Autodesk Inventor part; units mm, degrees
(part 2 of 3)
sketch "Sketch12" plane through (0, 0, 5) normal (0, 0, 1) x (1, 0, 0)
  circle A0 centre (-43.6086, -47.5396) radius 2.1 projected
  circle A1 centre (-50.585, -18.9546) radius 2.1 projected
  circle A2 centre (-57.5615, -47.5396) radius 2.1 projected
  circle A3 centre (-85.8051, -39.2889) radius 2.1 projected
  circle A4 centre (-64.538, -59.6232) radius 2.1 projected
  circle A5 centre (-85.8051, -79.9575) radius 2.1 projected
  circle A6 centre (-57.5615, -71.7068) radius 2.1 projected
  circle A7 centre (-50.585, -100.2918) radius 2.1 projected
  circle A8 centre (-43.6086, -71.7068) radius 2.1 projected
  circle A9 centre (-15.365, -79.9575) radius 2.1 projected
  circle A10 centre (-15.365, -39.2889) radius 2.1 projected
  circle A11 centre (-36.6321, -59.6232) radius 2.1 projected
  line L0 (-44.13, -38.9303) -> (-49.053, -44.7973) projected
  arc A12 (-52.1171, -44.7973) -> (-49.053, -44.7973) centre (-50.585, -43.5117) ccw projected
  line L1 (-52.1171, -44.7973) -> (-57.0401, -38.9303) projected
  arc A13 (-55.2842, -34.0514) -> (-57.0401, -38.9303) centre (-54.742, -37.0019) ccw projected
  arc A14 (-45.8859, -34.0514) -> (-55.2842, -34.0514) centre (-50.585, -59.6232) ccw projected
  arc A15 (-44.13, -38.9303) -> (-45.8859, -34.0514) centre (-46.4281, -37.0019) ccw projected
  line L2 (-65.2781, -43.6865) -> (-62.6586, -50.8834) projected
  arc A16 (-64.1907, -53.5371) -> (-62.6586, -50.8834) centre (-64.538, -51.5674) ccw projected
  line L3 (-64.1907, -53.5371) -> (-71.7331, -54.867) projected
  arc A17 (-75.0805, -50.9068) -> (-71.7331, -54.867) centre (-72.2541, -51.9126) ccw projected
  arc A18 (-70.3813, -42.7677) -> (-75.0805, -50.9068) centre (-50.585, -59.6232) ccw projected
  arc A19 (-65.2781, -43.6865) -> (-70.3813, -42.7677) centre (-68.0971, -44.7125) ccw projected
  line L4 (-71.7331, -64.3793) -> (-64.1907, -65.7093) projected
  arc A20 (-62.6586, -68.3629) -> (-64.1907, -65.7093) centre (-64.538, -67.6789) ccw projected
  line L5 (-62.6586, -68.3629) -> (-65.2781, -75.5599) projected
  arc A21 (-70.3813, -76.4787) -> (-65.2781, -75.5599) centre (-68.0971, -74.5338) ccw projected
  arc A22 (-75.0805, -68.3395) -> (-70.3813, -76.4787) centre (-50.585, -59.6232) ccw projected
  arc A23 (-71.7331, -64.3793) -> (-75.0805, -68.3395) centre (-72.2541, -67.3338) ccw projected
  line L6 (-57.0401, -80.316) -> (-52.1171, -74.449) projected
  arc A24 (-49.053, -74.449) -> (-52.1171, -74.449) centre (-50.585, -75.7346) ccw projected
  line L7 (-49.053, -74.449) -> (-44.13, -80.316) projected
  arc A25 (-45.8859, -85.195) -> (-44.13, -80.316) centre (-46.4281, -82.2444) ccw projected
  arc A26 (-55.2842, -85.195) -> (-45.8859, -85.195) centre (-50.585, -59.6232) ccw projected
  arc A27 (-57.0401, -80.316) -> (-55.2842, -85.195) centre (-54.742, -82.2444) ccw projected
  line L8 (-35.892, -75.5599) -> (-38.5115, -68.3629) projected
  arc A28 (-36.9794, -65.7093) -> (-38.5115, -68.3629) centre (-36.6321, -67.6789) ccw projected
  line L9 (-36.9794, -65.7093) -> (-29.437, -64.3793) projected
  arc A29 (-26.0896, -68.3395) -> (-29.437, -64.3793) centre (-28.916, -67.3338) ccw projected
  arc A30 (-30.7888, -76.4787) -> (-26.0896, -68.3395) centre (-50.585, -59.6232) ccw projected
  arc A31 (-35.892, -75.5599) -> (-30.7888, -76.4787) centre (-33.073, -74.5338) ccw projected
  line L10 (-29.437, -54.867) -> (-36.9794, -53.5371) projected
  arc A32 (-38.5115, -50.8834) -> (-36.9794, -53.5371) centre (-36.6321, -51.5674) ccw projected
  line L11 (-38.5115, -50.8834) -> (-35.892, -43.6865) projected
  arc A33 (-30.7888, -42.7677) -> (-35.892, -43.6865) centre (-33.073, -44.7125) ccw projected
  arc A34 (-26.0896, -50.9068) -> (-30.7888, -42.7677) centre (-50.585, -59.6232) ccw projected
  arc A35 (-29.437, -54.867) -> (-26.0896, -50.9068) centre (-28.916, -51.9126) ccw projected
  arc A36 (-83.4142, -91.845) -> (-62.0753, -104.165) centre (-50.585, -59.6232) ccw projected
  arc A37 (-83.0768, -85.9345) -> (-83.4142, -91.845) centre (-80.5595, -89.0431) ccw projected
  line L12 (-83.0768, -85.9345) -> (-78.075, -81.8841) projected
  arc A38 (-74.0235, -82.1373) -> (-78.075, -81.8841) centre (-76.1871, -84.2156) ccw projected
  arc A39 (-74.0235, -82.1373) -> (-58.3636, -91.1786) centre (-50.585, -59.6232) ccw projected
  arc A40 (-56.1186, -94.5607) -> (-58.3636, -91.1786) centre (-59.0817, -94.0914) ccw projected
  line L13 (-56.1186, -94.5607) -> (-57.1254, -100.9175) projected
  arc A41 (-62.0753, -104.165) -> (-57.1254, -100.9175) centre (-61.0762, -100.2918) ccw projected
  arc A42 (-39.0948, -104.165) -> (-17.7559, -91.845) centre (-50.585, -59.6232) ccw projected
  arc A43 (-44.0447, -100.9175) -> (-39.0948, -104.165) centre (-40.0939, -100.2918) ccw projected
  line L14 (-44.0447, -100.9175) -> (-45.0515, -94.5607) projected
  arc A44 (-42.8065, -91.1786) -> (-45.0515, -94.5607) centre (-42.0884, -94.0914) ccw projected
  arc A45 (-42.8065, -91.1786) -> (-27.1466, -82.1373) centre (-50.585, -59.6232) ccw projected
  arc A46 (-23.0951, -81.8841) -> (-27.1466, -82.1373) centre (-24.983, -84.2156) ccw projected
  line L15 (-23.0951, -81.8841) -> (-18.0933, -85.9345) projected
  arc A47 (-17.7559, -91.845) -> (-18.0933, -85.9345) centre (-20.6106, -89.0431) ccw projected
  arc A48 (-6.2656, -71.9432) -> (-6.2656, -47.3031) centre (-50.585, -59.6232) ccw projected
  arc A49 (-11.5529, -74.6062) -> (-6.2656, -71.9432) centre (-10.1194, -70.8719) ccw projected
  line L16 (-11.5529, -74.6062) -> (-17.5615, -72.2997) projected
  arc A50 (-19.368, -68.6644) -> (-17.5615, -72.2997) centre (-16.4864, -69.499) ccw projected
  arc A51 (-19.368, -68.6644) -> (-19.368, -50.5819) centre (-50.585, -59.6232) ccw projected
  arc A52 (-17.5615, -46.9466) -> (-19.368, -50.5819) centre (-16.4864, -49.7474) ccw projected
  line L17 (-17.5615, -46.9466) -> (-11.5529, -44.6401) projected
  arc A53 (-6.2656, -47.3031) -> (-11.5529, -44.6401) centre (-10.1194, -48.3745) ccw projected
  arc A54 (-17.7559, -27.4014) -> (-39.0948, -15.0814) centre (-50.585, -59.6232) ccw projected
  arc A55 (-18.0933, -33.3119) -> (-17.7559, -27.4014) centre (-20.6106, -30.2033) ccw projected
  line L18 (-18.0933, -33.3119) -> (-23.0951, -37.3622) projected
  arc A56 (-27.1466, -37.109) -> (-23.0951, -37.3622) centre (-24.983, -35.0308) ccw projected
  arc A57 (-27.1466, -37.109) -> (-42.8065, -28.0678) centre (-50.585, -59.6232) ccw projected
  arc A58 (-45.0515, -24.6857) -> (-42.8065, -28.0678) centre (-42.0884, -25.155) ccw projected
  line L19 (-45.0515, -24.6857) -> (-44.0447, -18.3288) projected
  arc A59 (-39.0948, -15.0814) -> (-44.0447, -18.3288) centre (-40.0939, -18.9546) ccw projected
  arc A60 (-62.0753, -15.0814) -> (-83.4142, -27.4014) centre (-50.585, -59.6232) ccw projected
  arc A61 (-57.1254, -18.3288) -> (-62.0753, -15.0814) centre (-61.0762, -18.9546) ccw projected
  line L20 (-57.1254, -18.3288) -> (-56.1186, -24.6857) projected
  arc A62 (-58.3636, -28.0678) -> (-56.1186, -24.6857) centre (-59.0817, -25.155) ccw projected
  arc A63 (-58.3636, -28.0678) -> (-74.0235, -37.109) centre (-50.585, -59.6232) ccw projected
  arc A64 (-78.075, -37.3622) -> (-74.0235, -37.109) centre (-76.1871, -35.0308) ccw projected
  line L21 (-78.075, -37.3622) -> (-83.0768, -33.3119) projected
  arc A65 (-83.4142, -27.4014) -> (-83.0768, -33.3119) centre (-80.5595, -30.2033) ccw projected
  arc A66 (-94.9045, -47.3031) -> (-94.9045, -71.9432) centre (-50.585, -59.6232) ccw projected
  arc A67 (-89.6172, -44.6401) -> (-94.9045, -47.3031) centre (-91.0507, -48.3745) ccw projected
  line L22 (-89.6172, -44.6401) -> (-83.6086, -46.9466) projected
  arc A68 (-81.8021, -50.5819) -> (-83.6086, -46.9466) centre (-84.6837, -49.7474) ccw projected
  arc A69 (-81.8021, -50.5819) -> (-81.8021, -68.6644) centre (-50.585, -59.6232) ccw projected
  arc A70 (-83.6086, -72.2997) -> (-81.8021, -68.6644) centre (-84.6837, -69.499) ccw projected
  line L23 (-83.6086, -72.2997) -> (-89.6172, -74.6062) projected
  arc A71 (-94.9045, -71.9432) -> (-89.6172, -74.6062) centre (-91.0507, -70.8719) ccw projected
  circle A72 centre (-36.0848, -126.8778) radius 16 projected
  circle A73 centre (-50.585, -59.6232) radius 8 projected
  circle A74 centre (4.8498, -18.875) radius 8 projected
  circle A75 centre (-26.0687, -154.0932) radius 1.5 projected
  circle A76 centre (-104.9663, -72.7226) radius 1.5 projected
  circle A77 centre (-102.1649, -37.0532) radius 1.5 projected
  circle A78 centre (14.3857, 5.6417) radius 1.5 projected
  circle A79 centre (13.3039, -43.7854) radius 1.5 projected
  circle A80 centre (31.1494, -18.2994) radius 1.5 projected
  circle A81 centre (-15.6668, -2.4109) radius 1.5 projected
  circle A82 centre (-91.1309, -21.0881) radius 1.5 projected
  circle A83 centre (-106.5395, -53.3794) radius 1.5 projected
  circle A84 centre (-53.3702, -150.5044) radius 1.5 projected
  circle A85 centre (-7.6073, -133.6622) radius 1.5 projected
  line L24 (-9.7265, -123.6247) -> (9.9725, -47.9268) projected
  line L25 (9.9725, -47.9268) -> (17.8509, -46.5376) projected
  line L26 (17.8509, -46.5376) -> (17.2063, -42.8816) projected
  arc A86 (17.2063, -42.8816) -> (31.6348, -22.2755) centre (4.8498, -18.875) ccw projected
  line L27 (31.6348, -22.2755) -> (35.2909, -21.6308) projected
  line L28 (35.2909, -21.6308) -> (33.9017, -13.7524) projected
  line L29 (33.9017, -13.7524) -> (27.008, -14.9679) projected
  arc A87 (27.008, -14.9679) -> (16.0998, 0.6106) centre (4.8498, -18.875) ccw projected
  line L30 (16.0998, 0.6106) -> (19.5998, 6.6727) projected
  line L31 (19.5998, 6.6727) -> (12.6716, 10.6727) projected
  line L32 (12.6716, 10.6727) -> (10.8154, 7.4577) projected
  arc A88 (10.8154, 7.4577) -> (-13.4829, 0.947) centre (4.8498, -18.875) ccw projected
  line L33 (-13.4829, 0.947) -> (-16.6979, 2.8032) projected
  line L34 (-16.6979, 2.8032) -> (-20.6979, -4.125) projected
  line L35 (-20.6979, -4.125) -> (-55.4348, -7.3477) projected
  arc A89 (-55.4348, -7.3477) -> (-76.835, -14.1568) centre (-50.585, -59.6232) ccw projected
  line L36 (-76.835, -14.1568) -> (-80.3713, -8.0318) projected
  line L37 (-80.3713, -8.0318) -> (-92.9509, -17.9357) projected
  arc A90 (-92.9509, -17.9357) -> (-96.423, -21.7867) centre (-50.585, -59.6232) ccw projected
  line L38 (-96.423, -21.7867) -> (-95.6743, -22.4047) projected
  arc A91 (-95.3624, -25.1669) -> (-95.6743, -22.4047) centre (-96.9475, -23.9472) ccw projected
  arc A92 (-95.3624, -25.1669) -> (-100.1355, -32.4754) centre (-50.585, -59.6232) ccw projected
  arc A93 (-102.79, -33.3003) -> (-100.1355, -32.4754) centre (-101.8895, -31.5145) ccw projected
  line L39 (-102.79, -33.3003) -> (-103.9829, -32.6988) projected
  arc A94 (-103.9829, -32.6988) -> (-106.5047, -38.4279) centre (-50.585, -59.6232) ccw projected
  line L40 (-106.5047, -38.4279) -> (-109.6106, -50.019) projected
  arc A95 (-109.6106, -50.019) -> (-110.2911, -56.2415) centre (-50.585, -59.6232) ccw projected
  line L41 (-110.2911, -56.2415) -> (-108.9573, -56.317) projected
  arc A96 (-107.0709, -58.3586) -> (-108.9573, -56.317) centre (-109.0704, -58.3138) ccw projected
  arc A97 (-107.0709, -58.3586) -> (-106.5915, -67.0745) centre (-50.585, -59.6232) ccw projected
  arc A98 (-108.2427, -69.3107) -> (-106.5915, -67.0745) centre (-108.5741, -67.3383) ccw projected
  line L42 (-108.2427, -69.3107) -> (-109.2001, -69.4715) projected
  arc A99 (-109.2001, -69.4715) -> (-108.1187, -74.5427) centre (-50.585, -59.6232) ccw projected
  line L43 (-108.1187, -74.5427) -> (-102.1764, -89.4094) projected
  line L44 (-102.1764, -89.4094) -> (-96.0514, -85.8732) projected
  arc A100 (-96.0514, -85.8732) -> (-93.2051, -90.2791) centre (-50.585, -59.6232) ccw projected
  line L45 (-93.2051, -90.2791) -> (-56.6733, -141.0681) projected
  arc A101 (-57.2313, -148.7428) -> (-56.6733, -141.0681) centre (-61.5442, -144.5716) ccw projected
  line L46 (-57.2313, -148.7428) -> (-59.0263, -150.5988) projected
  line L47 (-59.0263, -150.5988) -> (-54.7134, -154.77) projected
  line L48 (-54.7134, -154.77) -> (-51.8854, -154.7228) projected
  line L49 (-51.8854, -154.7228) -> (-50.3657, -153.1515) projected
  arc A102 (-48.0859, -152.7278) -> (-50.3657, -153.1515) centre (-48.9281, -154.5419) ccw projected
  arc A103 (-48.0859, -152.7278) -> (-31.6953, -155.0377) centre (-36.0848, -126.8778) ccw projected
  arc A104 (-29.5104, -156.3231) -> (-31.6953, -155.0377) centre (-31.3873, -157.0139) ccw projected
  line L50 (-29.5104, -156.3231) -> (-29.1318, -157.3516) projected
  line L51 (-29.1318, -157.3516) -> (-26.5641, -158.5378) projected
  line L52 (-26.5641, -158.5378) -> (-22.8103, -157.1563) projected
  line L53 (-22.8103, -157.1563) -> (-21.6241, -154.5886) projected
  line L54 (-21.6241, -154.5886) -> (-22.0027, -153.56) projected
  arc A105 (-21.1722, -151.1649) -> (-22.0027, -153.56) centre (-20.1257, -152.8693) ccw projected
  arc A106 (-21.1722, -151.1649) -> (-10.1895, -138.7808) centre (-36.0848, -126.8778) ccw projected
  arc A107 (-8.179, -137.6255) -> (-10.1895, -138.7808) centre (-8.3723, -139.6161) ccw projected
  line L55 (-8.179, -137.6255) -> (-6.0033, -137.8368) projected
  line L56 (-6.0033, -137.8368) -> (-3.8193, -136.0394) projected
  line L57 (-3.8193, -136.0394) -> (-3.2394, -130.0675) projected
  line L58 (-3.2394, -130.0675) -> (-5.371, -129.8605) projected
  arc A108 (-9.7265, -123.6247) -> (-5.371, -129.8605) centre (-4.8877, -124.8839) ccw projected
  circle A109 centre (-26.0687, -154.0932) radius 1.5 projected
  line L59 (-36.0848, -126.8778) -> (-26.0687, -154.0932)
  line L60 (-36.0848, -126.8778) -> (-45.311, -146.8497)
  circle A110 centre (-45.311, -146.8497) radius 2.05
  point P0 (0, 0)
  dimension "d80" = 22
  dimension "d81" = 45
  dimension "d82" = 4.1
  constraints: 4 end point, 1 centre point, 1 coincident
  measures "d80" distance of L59.start L60.end
  measures "d81" angle of L59 L60
  measures "d82" diameter of A110
extrude "Extrusion11" cut sketch "Sketch12" against normal blind 10 contours A110
pattern_circular "Circular Pattern6" count 4 over 360 about axis through (-36.0848, -126.8778, 5) along (0, 0, -1) of "Extrusion11"
sketch "Sketch13" plane through (0, 0, 5) normal (0, 0, 1) x (1, 0, 0)
  circle A0 centre (-16.1129, -136.1039) radius 2.05 projected
  circle A1 centre (-26.8587, -106.9059) radius 2.05 projected
  circle A2 centre (-56.0568, -117.6516) radius 2.05 projected
  circle A3 centre (-45.311, -146.8497) radius 2.05 projected
  circle A4 centre (-43.6086, -47.5396) radius 2.1 projected
  circle A5 centre (-50.585, -18.9546) radius 2.1 projected
  circle A6 centre (-57.5615, -47.5396) radius 2.1 projected
  circle A7 centre (-85.8051, -39.2889) radius 2.1 projected
  circle A8 centre (-64.538, -59.6232) radius 2.1 projected
  circle A9 centre (-85.8051, -79.9575) radius 2.1 projected
  circle A10 centre (-57.5615, -71.7068) radius 2.1 projected
  circle A11 centre (-50.585, -100.2918) radius 2.1 projected
  circle A12 centre (-43.6086, -71.7068) radius 2.1 projected
  circle A13 centre (-15.365, -79.9575) radius 2.1 projected
  circle A14 centre (-15.365, -39.2889) radius 2.1 projected
  circle A15 centre (-36.6321, -59.6232) radius 2.1 projected
  line L0 (-44.13, -38.9303) -> (-49.053, -44.7973) projected
  arc A16 (-52.1171, -44.7973) -> (-49.053, -44.7973) centre (-50.585, -43.5117) ccw projected
  line L1 (-52.1171, -44.7973) -> (-57.0401, -38.9303) projected
  arc A17 (-55.2842, -34.0514) -> (-57.0401, -38.9303) centre (-54.742, -37.0019) ccw projected
  arc A18 (-45.8859, -34.0514) -> (-55.2842, -34.0514) centre (-50.585, -59.6232) ccw projected
  arc A19 (-44.13, -38.9303) -> (-45.8859, -34.0514) centre (-46.4281, -37.0019) ccw projected
  line L2 (-65.2781, -43.6865) -> (-62.6586, -50.8834) projected
  arc A20 (-64.1907, -53.5371) -> (-62.6586, -50.8834) centre (-64.538, -51.5674) ccw projected
  line L3 (-64.1907, -53.5371) -> (-71.7331, -54.867) projected
  arc A21 (-75.0805, -50.9068) -> (-71.7331, -54.867) centre (-72.2541, -51.9126) ccw projected
  arc A22 (-70.3813, -42.7677) -> (-75.0805, -50.9068) centre (-50.585, -59.6232) ccw projected
  arc A23 (-65.2781, -43.6865) -> (-70.3813, -42.7677) centre (-68.0971, -44.7125) ccw projected
  line L4 (-71.7331, -64.3793) -> (-64.1907, -65.7093) projected
  arc A24 (-62.6586, -68.3629) -> (-64.1907, -65.7093) centre (-64.538, -67.6789) ccw projected
  line L5 (-62.6586, -68.3629) -> (-65.2781, -75.5599) projected
  arc A25 (-70.3813, -76.4787) -> (-65.2781, -75.5599) centre (-68.0971, -74.5338) ccw projected
  arc A26 (-75.0805, -68.3395) -> (-70.3813, -76.4787) centre (-50.585, -59.6232) ccw projected
  arc A27 (-71.7331, -64.3793) -> (-75.0805, -68.3395) centre (-72.2541, -67.3338) ccw projected
  line L6 (-57.0401, -80.316) -> (-52.1171, -74.449) projected
  arc A28 (-49.053, -74.449) -> (-52.1171, -74.449) centre (-50.585, -75.7346) ccw projected
  line L7 (-49.053, -74.449) -> (-44.13, -80.316) projected
  arc A29 (-45.8859, -85.195) -> (-44.13, -80.316) centre (-46.4281, -82.2444) ccw projected
  arc A30 (-55.2842, -85.195) -> (-45.8859, -85.195) centre (-50.585, -59.6232) ccw projected
  arc A31 (-57.0401, -80.316) -> (-55.2842, -85.195) centre (-54.742, -82.2444) ccw projected
  line L8 (-35.892, -75.5599) -> (-38.5115, -68.3629) projected
  arc A32 (-36.9794, -65.7093) -> (-38.5115, -68.3629) centre (-36.6321, -67.6789) ccw projected
  line L9 (-36.9794, -65.7093) -> (-29.437, -64.3793) projected
  arc A33 (-26.0896, -68.3395) -> (-29.437, -64.3793) centre (-28.916, -67.3338) ccw projected
  arc A34 (-30.7888, -76.4787) -> (-26.0896, -68.3395) centre (-50.585, -59.6232) ccw projected
  arc A35 (-35.892, -75.5599) -> (-30.7888, -76.4787) centre (-33.073, -74.5338) ccw projected
  line L10 (-29.437, -54.867) -> (-36.9794, -53.5371) projected
  arc A36 (-38.5115, -50.8834) -> (-36.9794, -53.5371) centre (-36.6321, -51.5674) ccw projected
  line L11 (-38.5115, -50.8834) -> (-35.892, -43.6865) projected
  arc A37 (-30.7888, -42.7677) -> (-35.892, -43.6865) centre (-33.073, -44.7125) ccw projected
  arc A38 (-26.0896, -50.9068) -> (-30.7888, -42.7677) centre (-50.585, -59.6232) ccw projected
  arc A39 (-29.437, -54.867) -> (-26.0896, -50.9068) centre (-28.916, -51.9126) ccw projected
  arc A40 (-83.4142, -91.845) -> (-62.0753, -104.165) centre (-50.585, -59.6232) ccw projected
  arc A41 (-83.0768, -85.9345) -> (-83.4142, -91.845) centre (-80.5595, -89.0431) ccw projected
  line L12 (-83.0768, -85.9345) -> (-78.075, -81.8841) projected
  arc A42 (-74.0235, -82.1373) -> (-78.075, -81.8841) centre (-76.1871, -84.2156) ccw projected
  arc A43 (-74.0235, -82.1373) -> (-58.3636, -91.1786) centre (-50.585, -59.6232) ccw projected
  arc A44 (-56.1186, -94.5607) -> (-58.3636, -91.1786) centre (-59.0817, -94.0914) ccw projected
  line L13 (-56.1186, -94.5607) -> (-57.1254, -100.9175) projected
  arc A45 (-62.0753, -104.165) -> (-57.1254, -100.9175) centre (-61.0762, -100.2918) ccw projected
  arc A46 (-39.0948, -104.165) -> (-17.7559, -91.845) centre (-50.585, -59.6232) ccw projected
  arc A47 (-44.0447, -100.9175) -> (-39.0948, -104.165) centre (-40.0939, -100.2918) ccw projected
  line L14 (-44.0447, -100.9175) -> (-45.0515, -94.5607) projected
  arc A48 (-42.8065, -91.1786) -> (-45.0515, -94.5607) centre (-42.0884, -94.0914) ccw projected
  arc A49 (-42.8065, -91.1786) -> (-27.1466, -82.1373) centre (-50.585, -59.6232) ccw projected
  arc A50 (-23.0951, -81.8841) -> (-27.1466, -82.1373) centre (-24.983, -84.2156) ccw projected
  line L15 (-23.0951, -81.8841) -> (-18.0933, -85.9345) projected
  arc A51 (-17.7559, -91.845) -> (-18.0933, -85.9345) centre (-20.6106, -89.0431) ccw projected
  arc A52 (-6.2656, -71.9432) -> (-6.2656, -47.3031) centre (-50.585, -59.6232) ccw projected
  arc A53 (-11.5529, -74.6062) -> (-6.2656, -71.9432) centre (-10.1194, -70.8719) ccw projected
  line L16 (-11.5529, -74.6062) -> (-17.5615, -72.2997) projected
  arc A54 (-19.368, -68.6644) -> (-17.5615, -72.2997) centre (-16.4864, -69.499) ccw projected
  arc A55 (-19.368, -68.6644) -> (-19.368, -50.5819) centre (-50.585, -59.6232) ccw projected
  arc A56 (-17.5615, -46.9466) -> (-19.368, -50.5819) centre (-16.4864, -49.7474) ccw projected
  line L17 (-17.5615, -46.9466) -> (-11.5529, -44.6401) projected
  arc A57 (-6.2656, -47.3031) -> (-11.5529, -44.6401) centre (-10.1194, -48.3745) ccw projected
  arc A58 (-17.7559, -27.4014) -> (-39.0948, -15.0814) centre (-50.585, -59.6232) ccw projected
  arc A59 (-18.0933, -33.3119) -> (-17.7559, -27.4014) centre (-20.6106, -30.2033) ccw projected
  line L18 (-18.0933, -33.3119) -> (-23.0951, -37.3622) projected
  arc A60 (-27.1466, -37.109) -> (-23.0951, -37.3622) centre (-24.983, -35.0308) ccw projected
  arc A61 (-27.1466, -37.109) -> (-42.8065, -28.0678) centre (-50.585, -59.6232) ccw projected
  arc A62 (-45.0515, -24.6857) -> (-42.8065, -28.0678) centre (-42.0884, -25.155) ccw projected
  line L19 (-45.0515, -24.6857) -> (-44.0447, -18.3288) projected
  arc A63 (-39.0948, -15.0814) -> (-44.0447, -18.3288) centre (-40.0939, -18.9546) ccw projected
  arc A64 (-62.0753, -15.0814) -> (-83.4142, -27.4014) centre (-50.585, -59.6232) ccw projected
  arc A65 (-57.1254, -18.3288) -> (-62.0753, -15.0814) centre (-61.0762, -18.9546) ccw projected
  line L20 (-57.1254, -18.3288) -> (-56.1186, -24.6857) projected
  arc A66 (-58.3636, -28.0678) -> (-56.1186, -24.6857) centre (-59.0817, -25.155) ccw projected
  arc A67 (-58.3636, -28.0678) -> (-74.0235, -37.109) centre (-50.585, -59.6232) ccw projected
  arc A68 (-78.075, -37.3622) -> (-74.0235, -37.109) centre (-76.1871, -35.0308) ccw projected
  line L21 (-78.075, -37.3622) -> (-83.0768, -33.3119) projected
  arc A69 (-83.4142, -27.4014) -> (-83.0768, -33.3119) centre (-80.5595, -30.2033) ccw projected
  arc A70 (-94.9045, -47.3031) -> (-94.9045, -71.9432) centre (-50.585, -59.6232) ccw projected
  arc A71 (-89.6172, -44.6401) -> (-94.9045, -47.3031) centre (-91.0507, -48.3745) ccw projected
  line L22 (-89.6172, -44.6401) -> (-83.6086, -46.9466) projected
  arc A72 (-81.8021, -50.5819) -> (-83.6086, -46.9466) centre (-84.6837, -49.7474) ccw projected
  arc A73 (-81.8021, -50.5819) -> (-81.8021, -68.6644) centre (-50.585, -59.6232) ccw projected
  arc A74 (-83.6086, -72.2997) -> (-81.8021, -68.6644) centre (-84.6837, -69.499) ccw projected
  line L23 (-83.6086, -72.2997) -> (-89.6172, -74.6062) projected
  arc A75 (-94.9045, -71.9432) -> (-89.6172, -74.6062) centre (-91.0507, -70.8719) ccw projected
  circle A76 centre (-36.0848, -126.8778) radius 16 projected
  circle A77 centre (-50.585, -59.6232) radius 8 projected
  circle A78 centre (4.8498, -18.875) radius 8 projected
  circle A79 centre (-26.0687, -154.0932) radius 1.5 projected
  circle A80 centre (-104.9663, -72.7226) radius 1.5 projected
  circle A81 centre (-102.1649, -37.0532) radius 1.5 projected
  circle A82 centre (14.3857, 5.6417) radius 1.5 projected
  circle A83 centre (13.3039, -43.7854) radius 1.5 projected
  circle A84 centre (31.1494, -18.2994) radius 1.5 projected
  circle A85 centre (-15.6668, -2.4109) radius 1.5 projected
  circle A86 centre (-91.1309, -21.0881) radius 1.5 projected
  circle A87 centre (-106.5395, -53.3794) radius 1.5 projected
  circle A88 centre (-53.3702, -150.5044) radius 1.5 projected
  circle A89 centre (-7.6073, -133.6622) radius 1.5 projected
  line L24 (-9.7265, -123.6247) -> (9.9725, -47.9268) projected
  line L25 (9.9725, -47.9268) -> (17.8509, -46.5376) projected
  line L26 (17.8509, -46.5376) -> (17.2063, -42.8816) projected
  arc A90 (17.2063, -42.8816) -> (31.6348, -22.2755) centre (4.8498, -18.875) ccw projected
  line L27 (31.6348, -22.2755) -> (35.2909, -21.6308) projected
  line L28 (35.2909, -21.6308) -> (33.9017, -13.7524) projected
  line L29 (33.9017, -13.7524) -> (27.008, -14.9679) projected
  arc A91 (27.008, -14.9679) -> (16.0998, 0.6106) centre (4.8498, -18.875) ccw projected
  line L30 (16.0998, 0.6106) -> (19.5998, 6.6727) projected
  line L31 (19.5998, 6.6727) -> (12.6716, 10.6727) projected
  line L32 (12.6716, 10.6727) -> (10.8154, 7.4577) projected
  arc A92 (10.8154, 7.4577) -> (-13.4829, 0.947) centre (4.8498, -18.875) ccw projected
  line L33 (-13.4829, 0.947) -> (-16.6979, 2.8032) projected
  line L34 (-16.6979, 2.8032) -> (-20.6979, -4.125) projected
  line L35 (-20.6979, -4.125) -> (-55.4348, -7.3477) projected
  arc A93 (-55.4348, -7.3477) -> (-76.835, -14.1568) centre (-50.585, -59.6232) ccw projected
  line L36 (-76.835, -14.1568) -> (-80.3713, -8.0318) projected
  line L37 (-80.3713, -8.0318) -> (-92.9509, -17.9357) projected
  arc A94 (-92.9509, -17.9357) -> (-96.423, -21.7867) centre (-50.585, -59.6232) ccw projected
  line L38 (-96.423, -21.7867) -> (-95.6743, -22.4047) projected
  arc A95 (-95.3624, -25.1669) -> (-95.6743, -22.4047) centre (-96.9475, -23.9472) ccw projected
  arc A96 (-95.3624, -25.1669) -> (-100.1355, -32.4754) centre (-50.585, -59.6232) ccw projected
  arc A97 (-102.79, -33.3003) -> (-100.1355, -32.4754) centre (-101.8895, -31.5145) ccw projected
  line L39 (-102.79, -33.3003) -> (-103.9829, -32.6988) projected
  arc A98 (-103.9829, -32.6988) -> (-106.5047, -38.4279) centre (-50.585, -59.6232) ccw projected
  line L40 (-106.5047, -38.4279) -> (-109.6106, -50.019) projected
  arc A99 (-109.6106, -50.019) -> (-110.2911, -56.2415) centre (-50.585, -59.6232) ccw projected
  line L41 (-110.2911, -56.2415) -> (-108.9573, -56.317) projected
  arc A100 (-107.0709, -58.3586) -> (-108.9573, -56.317) centre (-109.0704, -58.3138) ccw projected
  arc A101 (-107.0709, -58.3586) -> (-106.5915, -67.0745) centre (-50.585, -59.6232) ccw projected
  arc A102 (-108.2427, -69.3107) -> (-106.5915, -67.0745) centre (-108.5741, -67.3383) ccw projected
  line L42 (-108.2427, -69.3107) -> (-109.2001, -69.4715) projected
  arc A103 (-109.2001, -69.4715) -> (-108.1187, -74.5427) centre (-50.585, -59.6232) ccw projected
  line L43 (-108.1187, -74.5427) -> (-102.1764, -89.4094) projected
  line L44 (-102.1764, -89.4094) -> (-96.0514, -85.8732) projected
  arc A104 (-96.0514, -85.8732) -> (-93.2051, -90.2791) centre (-50.585, -59.6232) ccw projected
  line L45 (-93.2051, -90.2791) -> (-56.6733, -141.0681) projected
  arc A105 (-57.2313, -148.7428) -> (-56.6733, -141.0681) centre (-61.5442, -144.5716) ccw projected
  line L46 (-57.2313, -148.7428) -> (-59.0263, -150.5988) projected
  line L47 (-59.0263, -150.5988) -> (-54.7134, -154.77) projected
  line L48 (-54.7134, -154.77) -> (-51.8854, -154.7228) projected
  line L49 (-51.8854, -154.7228) -> (-50.3657, -153.1515) projected
  arc A106 (-48.0859, -152.7278) -> (-50.3657, -153.1515) centre (-48.9281, -154.5419) ccw projected
  arc A107 (-48.0859, -152.7278) -> (-31.6953, -155.0377) centre (-36.0848, -126.8778) ccw projected
  arc A108 (-29.5104, -156.3231) -> (-31.6953, -155.0377) centre (-31.3873, -157.0139) ccw projected
  line L50 (-29.5104, -156.3231) -> (-29.1318, -157.3516) projected
  line L51 (-29.1318, -157.3516) -> (-26.5641, -158.5378) projected
  line L52 (-26.5641, -158.5378) -> (-22.8103, -157.1563) projected
  line L53 (-22.8103, -157.1563) -> (-21.6241, -154.5886) projected
  line L54 (-21.6241, -154.5886) -> (-22.0027, -153.56) projected
  arc A109 (-21.1722, -151.1649) -> (-22.0027, -153.56) centre (-20.1257, -152.8693) ccw projected
  arc A110 (-21.1722, -151.1649) -> (-10.1895, -138.7808) centre (-36.0848, -126.8778) ccw projected
  arc A111 (-8.179, -137.6255) -> (-10.1895, -138.7808) centre (-8.3723, -139.6161) ccw projected
  line L55 (-8.179, -137.6255) -> (-6.0033, -137.8368) projected
  line L56 (-6.0033, -137.8368) -> (-3.8193, -136.0394) projected
  line L57 (-3.8193, -136.0394) -> (-3.2394, -130.0675) projected
  line L58 (-3.2394, -130.0675) -> (-5.371, -129.8605) projected
  arc A112 (-9.7265, -123.6247) -> (-5.371, -129.8605) centre (-4.8877, -124.8839) ccw projected
  line L59 (-14.8426, -119.4603) -> (-6.4101, -87.0562)
  circle A113 centre (-36.0848, -126.8778) radius 22.5
  circle A114 centre (-50.585, -59.6232) radius 52
  line L60 (-20.7537, -110.4094) -> (-18.1052, -100.2318)
  line L61 (-58.5466, -128.1884) -> (-74.7431, -105.6708)
  circle A115 centre (-36.0848, -126.8778) radius 27.5
  point P0 (0, 0)
  point P1 (-63.1181, -121.8328)
  point P2 (-58.5453, -111.0103)
  point P3 (-19.3588, -105.0491)
  point P4 (-12.9173, -112.0618)
  dimension "d88" = 45
  dimension "d89" = 6
  dimension "d90" = 104
  dimension "d91" = 8
  dimension "d92" = 6
  dimension "d93" = 55
  constraints: 6 end point, 6 point on circle, 3 centre point, 3 coincident, 3 parallel
  measures "d88" diameter of A113
  measures "d89" distance between parallel lines of L24 L59
  measures "d90" diameter of A114
  measures "d91" distance between parallel lines of L59 L60
  measures "d92" distance between parallel lines of L45 L61
  measures "d93" diameter of A115
extrude "Extrusion12" cut sketch "Sketch13" against normal blind 10 contours A115 L60 A114 L59 | L61 A114 A115
fillet "Fillet12" radius 2 5 edges at (-6.4101, -87.0562, 2.5) (-12.9173, -112.0618, 2.5) (-74.7431, -105.6708, 2.5) (-63.1181, -121.8328, 2.5) (-58.5453, -111.0103, 2.5)
fillet "Fillet13" radius 3 1 edges at (-19.3588, -105.0491, 2.5)
fillet "Fillet14" radius 5 1 edges at (-18.1052, -100.2318, 2.5)
thicken "Thicken1" operation add thickness 3 both sides no extend neighbours yes toward (-0.745193, -0.6668488, 0) faces at (-15.592, -108.5394, 1.6667)
sketch "Sketch14" plane through (0, 0, 5) normal (0, 0, 1) x (1, 0, 0)
  circle A0 centre (2.1523, -31.0805) radius 2.1 projected
  circle A1 centre (17.0553, -21.5725) radius 2.1 projected
  circle A2 centre (7.5473, -6.6695) radius 2.1 projected
  circle A3 centre (-7.3556, -16.1775) radius 2.1 projected
  point P0 (0, 0)
hole "Hole3" at (17.0553, -21.5725, 5) at (2.1523, -31.0805, 5) at (-7.3556, -16.1775, 5) at (7.5473, -6.6695, 5) direction (0, 0, -1) diameter 3.1 depth 17
sketch "Sketch15" plane through (0, 0, 5) normal (0, 0, 1) x (1, 0, 0)
  circle A0 centre (-7.3556, -16.1775) radius 1.55 projected
  circle A1 centre (17.0553, -21.5725) radius 1.55 projected
  circle A2 centre (2.1523, -31.0805) radius 1.55 projected
  circle A3 centre (7.5473, -6.6695) radius 1.55 projected
  line L0 (-8.9194, -96.699) -> (-12.8137, -111.6638) projected
  arc A4 (-16.3595, -112.3464) -> (-12.8137, -111.6638) centre (-14.7493, -111.1602) ccw projected
  arc A5 (-16.3595, -112.3464) -> (-18.9305, -109.3855) centre (-36.0848, -126.8778) ccw projected
  arc A6 (-19.7333, -106.4881) -> (-18.9305, -109.3855) centre (-16.83, -107.2436) ccw projected
  line L1 (-19.7333, -106.4881) -> (-18.513, -101.7988) projected
  arc A7 (-16.9119, -99.2479) -> (-18.513, -101.7988) centre (-13.6742, -103.058) ccw projected
  arc A8 (-16.9119, -99.2479) -> (-12.3264, -94.8408) centre (-50.585, -59.6232) ccw projected
  arc A9 (-8.9194, -96.699) -> (-12.3264, -94.8408) centre (-10.8549, -96.1953) ccw projected
  arc A10 (-68.172, -108.5588) -> (-61.3963, -110.4869) centre (-50.585, -59.6232) ccw projected
  arc A11 (-60.0679, -113.4218) -> (-61.3963, -110.4869) centre (-61.8121, -112.4432) ccw projected
  arc A12 (-60.0679, -113.4218) -> (-62.0734, -117.8863) centre (-36.0848, -126.8778) ccw projected
  arc A13 (-65.5871, -118.4003) -> (-62.0734, -117.8863) centre (-63.9634, -117.2324) ccw projected
  line L2 (-65.5871, -118.4003) -> (-70.472, -111.6088) projected
  arc A14 (-68.172, -108.5588) -> (-70.472, -111.6088) centre (-68.8484, -110.441) ccw projected
  circle A15 centre (-16.1129, -136.1039) radius 2.05 projected
  circle A16 centre (-26.8587, -106.9059) radius 2.05 projected
  circle A17 centre (-56.0568, -117.6516) radius 2.05 projected
  circle A18 centre (-45.311, -146.8497) radius 2.05 projected
  circle A19 centre (-43.6086, -47.5396) radius 2.1 projected
  circle A20 centre (-50.585, -18.9546) radius 2.1 projected
  circle A21 centre (-57.5615, -47.5396) radius 2.1 projected
  circle A22 centre (-85.8051, -39.2889) radius 2.1 projected
  circle A23 centre (-64.538, -59.6232) radius 2.1 projected
  circle A24 centre (-85.8051, -79.9575) radius 2.1 projected
  circle A25 centre (-57.5615, -71.7068) radius 2.1 projected
  circle A26 centre (-50.585, -100.2918) radius 2.1 projected
  circle A27 centre (-43.6086, -71.7068) radius 2.1 projected
  circle A28 centre (-15.365, -79.9575) radius 2.1 projected
  circle A29 centre (-15.365, -39.2889) radius 2.1 projected
  circle A30 centre (-36.6321, -59.6232) radius 2.1 projected
  line L3 (-44.13, -38.9303) -> (-49.053, -44.7973) projected
  arc A31 (-52.1171, -44.7973) -> (-49.053, -44.7973) centre (-50.585, -43.5117) ccw projected
  line L4 (-52.1171, -44.7973) -> (-57.0401, -38.9303) projected
  arc A32 (-55.2842, -34.0514) -> (-57.0401, -38.9303) centre (-54.742, -37.0019) ccw projected
  arc A33 (-45.8859, -34.0514) -> (-55.2842, -34.0514) centre (-50.585, -59.6232) ccw projected
  arc A34 (-44.13, -38.9303) -> (-45.8859, -34.0514) centre (-46.4281, -37.0019) ccw projected
  line L5 (-65.2781, -43.6865) -> (-62.6586, -50.8834) projected
  arc A35 (-64.1907, -53.5371) -> (-62.6586, -50.8834) centre (-64.538, -51.5674) ccw projected
  line L6 (-64.1907, -53.5371) -> (-71.7331, -54.867) projected
  arc A36 (-75.0805, -50.9068) -> (-71.7331, -54.867) centre (-72.2541, -51.9126) ccw projected
  arc A37 (-70.3813, -42.7677) -> (-75.0805, -50.9068) centre (-50.585, -59.6232) ccw projected
  arc A38 (-65.2781, -43.6865) -> (-70.3813, -42.7677) centre (-68.0971, -44.7125) ccw projected
  line L7 (-71.7331, -64.3793) -> (-64.1907, -65.7093) projected
  arc A39 (-62.6586, -68.3629) -> (-64.1907, -65.7093) centre (-64.538, -67.6789) ccw projected
  line L8 (-62.6586, -68.3629) -> (-65.2781, -75.5599) projected
  arc A40 (-70.3813, -76.4787) -> (-65.2781, -75.5599) centre (-68.0971, -74.5338) ccw projected
  arc A41 (-75.0805, -68.3395) -> (-70.3813, -76.4787) centre (-50.585, -59.6232) ccw projected
  arc A42 (-71.7331, -64.3793) -> (-75.0805, -68.3395) centre (-72.2541, -67.3338) ccw projected
  line L9 (-57.0401, -80.316) -> (-52.1171, -74.449) projected
  arc A43 (-49.053, -74.449) -> (-52.1171, -74.449) centre (-50.585, -75.7346) ccw projected
  line L10 (-49.053, -74.449) -> (-44.13, -80.316) projected
  arc A44 (-45.8859, -85.195) -> (-44.13, -80.316) centre (-46.4281, -82.2444) ccw projected
  arc A45 (-55.2842, -85.195) -> (-45.8859, -85.195) centre (-50.585, -59.6232) ccw projected
  arc A46 (-57.0401, -80.316) -> (-55.2842, -85.195) centre (-54.742, -82.2444) ccw projected
  line L11 (-35.892, -75.5599) -> (-38.5115, -68.3629) projected
  arc A47 (-36.9794, -65.7093) -> (-38.5115, -68.3629) centre (-36.6321, -67.6789) ccw projected
  line L12 (-36.9794, -65.7093) -> (-29.437, -64.3793) projected
  arc A48 (-26.0896, -68.3395) -> (-29.437, -64.3793) centre (-28.916, -67.3338) ccw projected
  arc A49 (-30.7888, -76.4787) -> (-26.0896, -68.3395) centre (-50.585, -59.6232) ccw projected
  arc A50 (-35.892, -75.5599) -> (-30.7888, -76.4787) centre (-33.073, -74.5338) ccw projected
  line L13 (-29.437, -54.867) -> (-36.9794, -53.5371) projected
  arc A51 (-38.5115, -50.8834) -> (-36.9794, -53.5371) centre (-36.6321, -51.5674) ccw projected
  line L14 (-38.5115, -50.8834) -> (-35.892, -43.6865) projected
  arc A52 (-30.7888, -42.7677) -> (-35.892, -43.6865) centre (-33.073, -44.7125) ccw projected
  arc A53 (-26.0896, -50.9068) -> (-30.7888, -42.7677) centre (-50.585, -59.6232) ccw projected
  arc A54 (-29.437, -54.867) -> (-26.0896, -50.9068) centre (-28.916, -51.9126) ccw projected
  arc A55 (-83.4142, -91.845) -> (-62.0753, -104.165) centre (-50.585, -59.6232) ccw projected
  arc A56 (-83.0768, -85.9345) -> (-83.4142, -91.845) centre (-80.5595, -89.0431) ccw projected
  line L15 (-83.0768, -85.9345) -> (-78.075, -81.8841) projected
  arc A57 (-74.0235, -82.1373) -> (-78.075, -81.8841) centre (-76.1871, -84.2156) ccw projected
  arc A58 (-74.0235, -82.1373) -> (-58.3636, -91.1786) centre (-50.585, -59.6232) ccw projected
  arc A59 (-56.1186, -94.5607) -> (-58.3636, -91.1786) centre (-59.0817, -94.0914) ccw projected
  line L16 (-56.1186, -94.5607) -> (-57.1254, -100.9175) projected
  arc A60 (-62.0753, -104.165) -> (-57.1254, -100.9175) centre (-61.0762, -100.2918) ccw projected
  arc A61 (-39.0948, -104.165) -> (-17.7559, -91.845) centre (-50.585, -59.6232) ccw projected
  arc A62 (-44.0447, -100.9175) -> (-39.0948, -104.165) centre (-40.0939, -100.2918) ccw projected
  line L17 (-44.0447, -100.9175) -> (-45.0515, -94.5607) projected
  arc A63 (-42.8065, -91.1786) -> (-45.0515, -94.5607) centre (-42.0884, -94.0914) ccw projected
  arc A64 (-42.8065, -91.1786) -> (-27.1466, -82.1373) centre (-50.585, -59.6232) ccw projected
  arc A65 (-23.0951, -81.8841) -> (-27.1466, -82.1373) centre (-24.983, -84.2156) ccw projected
  line L18 (-23.0951, -81.8841) -> (-18.0933, -85.9345) projected
  arc A66 (-17.7559, -91.845) -> (-18.0933, -85.9345) centre (-20.6106, -89.0431) ccw projected
  arc A67 (-6.2656, -71.9432) -> (-6.2656, -47.3031) centre (-50.585, -59.6232) ccw projected
  arc A68 (-11.5529, -74.6062) -> (-6.2656, -71.9432) centre (-10.1194, -70.8719) ccw projected
  line L19 (-11.5529, -74.6062) -> (-17.5615, -72.2997) projected
  arc A69 (-19.368, -68.6644) -> (-17.5615, -72.2997) centre (-16.4864, -69.499) ccw projected
  arc A70 (-19.368, -68.6644) -> (-19.368, -50.5819) centre (-50.585, -59.6232) ccw projected
  arc A71 (-17.5615, -46.9466) -> (-19.368, -50.5819) centre (-16.4864, -49.7474) ccw projected
  line L20 (-17.5615, -46.9466) -> (-11.5529, -44.6401) projected
  arc A72 (-6.2656, -47.3031) -> (-11.5529, -44.6401) centre (-10.1194, -48.3745) ccw projected
  arc A73 (-17.7559, -27.4014) -> (-39.0948, -15.0814) centre (-50.585, -59.6232) ccw projected
  arc A74 (-18.0933, -33.3119) -> (-17.7559, -27.4014) centre (-20.6106, -30.2033) ccw projected
  line L21 (-18.0933, -33.3119) -> (-23.0951, -37.3622) projected
  arc A75 (-27.1466, -37.109) -> (-23.0951, -37.3622) centre (-24.983, -35.0308) ccw projected
  arc A76 (-27.1466, -37.109) -> (-42.8065, -28.0678) centre (-50.585, -59.6232) ccw projected
  arc A77 (-45.0515, -24.6857) -> (-42.8065, -28.0678) centre (-42.0884, -25.155) ccw projected
  line L22 (-45.0515, -24.6857) -> (-44.0447, -18.3288) projected
  arc A78 (-39.0948, -15.0814) -> (-44.0447, -18.3288) centre (-40.0939, -18.9546) ccw projected
  arc A79 (-62.0753, -15.0814) -> (-83.4142, -27.4014) centre (-50.585, -59.6232) ccw projected
  arc A80 (-57.1254, -18.3288) -> (-62.0753, -15.0814) centre (-61.0762, -18.9546) ccw projected
  line L23 (-57.1254, -18.3288) -> (-56.1186, -24.6857) projected
  arc A81 (-58.3636, -28.0678) -> (-56.1186, -24.6857) centre (-59.0817, -25.155) ccw projected
  arc A82 (-58.3636, -28.0678) -> (-74.0235, -37.109) centre (-50.585, -59.6232) ccw projected
  arc A83 (-78.075, -37.3622) -> (-74.0235, -37.109) centre (-76.1871, -35.0308) ccw projected
  line L24 (-78.075, -37.3622) -> (-83.0768, -33.3119) projected
  arc A84 (-83.4142, -27.4014) -> (-83.0768, -33.3119) centre (-80.5595, -30.2033) ccw projected
  arc A85 (-94.9045, -47.3031) -> (-94.9045, -71.9432) centre (-50.585, -59.6232) ccw projected
  arc A86 (-89.6172, -44.6401) -> (-94.9045, -47.3031) centre (-91.0507, -48.3745) ccw projected
  line L25 (-89.6172, -44.6401) -> (-83.6086, -46.9466) projected
  arc A87 (-81.8021, -50.5819) -> (-83.6086, -46.9466) centre (-84.6837, -49.7474) ccw projected
  arc A88 (-81.8021, -50.5819) -> (-81.8021, -68.6644) centre (-50.585, -59.6232) ccw projected
  arc A89 (-83.6086, -72.2997) -> (-81.8021, -68.6644) centre (-84.6837, -69.499) ccw projected
  line L26 (-83.6086, -72.2997) -> (-89.6172, -74.6062) projected
  arc A90 (-94.9045, -71.9432) -> (-89.6172, -74.6062) centre (-91.0507, -70.8719) ccw projected
  circle A91 centre (-36.0848, -126.8778) radius 16 projected
  circle A92 centre (-50.585, -59.6232) radius 8 projected
  circle A93 centre (4.8498, -18.875) radius 8 projected
  circle A94 centre (-26.0687, -154.0932) radius 1.5 projected
  circle A95 centre (-104.9663, -72.7226) radius 1.5 projected
  circle A96 centre (-102.1649, -37.0532) radius 1.5 projected
  circle A97 centre (14.3857, 5.6417) radius 1.5 projected
  circle A98 centre (13.3039, -43.7854) radius 1.5 projected
  circle A99 centre (31.1494, -18.2994) radius 1.5 projected
  circle A100 centre (-15.6668, -2.4109) radius 1.5 projected
  circle A101 centre (-91.1309, -21.0881) radius 1.5 projected
  circle A102 centre (-106.5395, -53.3794) radius 1.5 projected
  circle A103 centre (-53.3702, -150.5044) radius 1.5 projected
  circle A104 centre (-7.6073, -133.6622) radius 1.5 projected
  line L27 (-9.7265, -123.6247) -> (9.9725, -47.9268) projected
  line L28 (9.9725, -47.9268) -> (17.8509, -46.5376) projected
  line L29 (17.8509, -46.5376) -> (17.2063, -42.8816) projected
  arc A105 (17.2063, -42.8816) -> (31.6348, -22.2755) centre (4.8498, -18.875) ccw projected
  line L30 (31.6348, -22.2755) -> (35.2909, -21.6308) projected
  line L31 (35.2909, -21.6308) -> (33.9017, -13.7524) projected
  line L32 (33.9017, -13.7524) -> (27.008, -14.9679) projected
  arc A106 (27.008, -14.9679) -> (16.0998, 0.6106) centre (4.8498, -18.875) ccw projected
  line L33 (16.0998, 0.6106) -> (19.5998, 6.6727) projected
  line L34 (19.5998, 6.6727) -> (12.6716, 10.6727) projected
  line L35 (12.6716, 10.6727) -> (10.8154, 7.4577) projected
  arc A107 (10.8154, 7.4577) -> (-13.4829, 0.947) centre (4.8498, -18.875) ccw projected
  line L36 (-13.4829, 0.947) -> (-16.6979, 2.8032) projected
  line L37 (-16.6979, 2.8032) -> (-20.6979, -4.125) projected
  line L38 (-20.6979, -4.125) -> (-55.4348, -7.3477) projected
  arc A108 (-55.4348, -7.3477) -> (-76.835, -14.1568) centre (-50.585, -59.6232) ccw projected
  line L39 (-76.835, -14.1568) -> (-80.3713, -8.0318) projected
  line L40 (-80.3713, -8.0318) -> (-92.9509, -17.9357) projected
  arc A109 (-92.9509, -17.9357) -> (-96.423, -21.7867) centre (-50.585, -59.6232) ccw projected
  line L41 (-96.423, -21.7867) -> (-95.6743, -22.4047) projected
  arc A110 (-95.3624, -25.1669) -> (-95.6743, -22.4047) centre (-96.9475, -23.9472) ccw projected
  arc A111 (-95.3624, -25.1669) -> (-100.1355, -32.4754) centre (-50.585, -59.6232) ccw projected
  arc A112 (-102.79, -33.3003) -> (-100.1355, -32.4754) centre (-101.8895, -31.5145) ccw projected
  line L42 (-102.79, -33.3003) -> (-103.9829, -32.6988) projected
  arc A113 (-103.9829, -32.6988) -> (-106.5047, -38.4279) centre (-50.585, -59.6232) ccw projected
  line L43 (-106.5047, -38.4279) -> (-109.6106, -50.019) projected
  arc A114 (-109.6106, -50.019) -> (-110.2911, -56.2415) centre (-50.585, -59.6232) ccw projected
  line L44 (-110.2911, -56.2415) -> (-108.9573, -56.317) projected
  arc A115 (-107.0709, -58.3586) -> (-108.9573, -56.317) centre (-109.0704, -58.3138) ccw projected
  arc A116 (-107.0709, -58.3586) -> (-106.5915, -67.0745) centre (-50.585, -59.6232) ccw projected
  arc A117 (-108.2427, -69.3107) -> (-106.5915, -67.0745) centre (-108.5741, -67.3383) ccw projected
  line L45 (-108.2427, -69.3107) -> (-109.2001, -69.4715) projected
  arc A118 (-109.2001, -69.4715) -> (-108.1187, -74.5427) centre (-50.585, -59.6232) ccw projected
  line L46 (-108.1187, -74.5427) -> (-102.1764, -89.4094) projected
  line L47 (-102.1764, -89.4094) -> (-96.0514, -85.8732) projected
  arc A119 (-96.0514, -85.8732) -> (-93.2051, -90.2791) centre (-50.585, -59.6232) ccw projected
  line L48 (-93.2051, -90.2791) -> (-56.6733, -141.0681) projected
  arc A120 (-57.2313, -148.7428) -> (-56.6733, -141.0681) centre (-61.5442, -144.5716) ccw projected
  line L49 (-57.2313, -148.7428) -> (-59.0263, -150.5988) projected
  line L50 (-59.0263, -150.5988) -> (-54.7134, -154.77) projected
  line L51 (-54.7134, -154.77) -> (-51.8854, -154.7228) projected
  line L52 (-51.8854, -154.7228) -> (-50.3657, -153.1515) projected
  arc A121 (-48.0859, -152.7278) -> (-50.3657, -153.1515) centre (-48.9281, -154.5419) ccw projected
  arc A122 (-48.0859, -152.7278) -> (-31.6953, -155.0377) centre (-36.0848, -126.8778) ccw projected
  arc A123 (-29.5104, -156.3231) -> (-31.6953, -155.0377) centre (-31.3873, -157.0139) ccw projected
  line L53 (-29.5104, -156.3231) -> (-29.1318, -157.3516) projected
  line L54 (-29.1318, -157.3516) -> (-26.5641, -158.5378) projected
  line L55 (-26.5641, -158.5378) -> (-22.8103, -157.1563) projected
  line L56 (-22.8103, -157.1563) -> (-21.6241, -154.5886) projected
  line L57 (-21.6241, -154.5886) -> (-22.0027, -153.56) projected
  arc A124 (-21.1722, -151.1649) -> (-22.0027, -153.56) centre (-20.1257, -152.8693) ccw projected
  arc A125 (-21.1722, -151.1649) -> (-10.1895, -138.7808) centre (-36.0848, -126.8778) ccw projected
  arc A126 (-8.179, -137.6255) -> (-10.1895, -138.7808) centre (-8.3723, -139.6161) ccw projected
  line L58 (-8.179, -137.6255) -> (-6.0033, -137.8368) projected
  line L59 (-6.0033, -137.8368) -> (-3.8193, -136.0394) projected
  line L60 (-3.8193, -136.0394) -> (-3.2394, -130.0675) projected
  line L61 (-3.2394, -130.0675) -> (-5.371, -129.8605) projected
  arc A127 (-9.7265, -123.6247) -> (-5.371, -129.8605) centre (-4.8877, -124.8839) ccw projected
  line L62 (7.5473, -6.6695) -> (17.0553, -21.5725)
  line L63 (4.8498, -18.875) -> (12.3013, -14.121)
  line L64 (12.3013, -14.121) -> (15.6735, -11.9696)
  circle A128 centre (15.6735, -11.9696) radius 2.05
  point P0 (0, 0)
  dimension "d108" = 4
  dimension "d109" = 4.1
  constraints: 6 end point, 1 centre point, 1 coincident, 1 midpoint, 1 perpendicular
  measures "d108" distance of L63.end L64.end
  measures "d109" diameter of A128
extrude "Extrusion13" cut sketch "Sketch15" against normal blind 10 contours A128
pattern_circular "Circular Pattern7" count 4 over 360 about axis through (4.8498, -18.875, 5) along (0, 0, -1) of "Extrusion13"